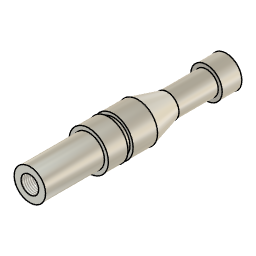
MSE 480 Lab 2 v4 (Autodesk Fusion 360 design; units mm, degrees)
Autodesk Fusion 360 part; units mm, degrees
note: some values were not read from the file. Chosen so that the rebuilt part matches the saved one: that a step has no effect; how an offset face is resized. Set by a fixed rule: which sketch regions a step uses.
sketch "Sketch2" plane through (0, 0, 0) normal (1, 0, 0) x (0, 1, 0)
  line L0 (0, 10.16) -> (38.1, 10.16)
  line L1 (38.1, 10.16) -> (38.1, 12.7)
  line L2 (38.1, 12.7) -> (50.8, 12.7)
  line L3 (50.8, 12.7) -> (50.8, 10.668)
  line L4 (50.8, 10.668) -> (54.102, 10.668)
  line L5 (54.102, 10.668) -> (54.102, 12.7)
  line L6 (54.102, 12.7) -> (69.9412, 12.7)
  line L7 (0, 10.16) -> (0, 0)
  line L8 (127, 0) -> (127, 10.16)
  line L9 (127, 10.16) -> (114.3, 10.16)
  line L10 (114.3, 10.16) -> (114.3, 7.62)
  line L11 (114.3, 7.62) -> (88.9, 7.62)
  line L12 (88.9, 7.62) -> (69.9412, 12.7)
  line L13 (0, 0) -> (127, 0)
  dimension "d4" = 3.302
  dimension "d5" = 12.7
  dimension "d6" = 38.1
  dimension "d14" = 127
  dimension "d15" = 25.4
  dimension "d16" = 12.7
  dimension "d17" = 2.54
  dimension "d30" = 165
  dimension "d64" = 10.16
  dimension "d65" = 10.16
  dimension "d72" = 2.032
  dimension "d73" = 2.54
  dimension "d74" = 7.62
  constraint perpendicular L0 L1
  constraint perpendicular L1 L2
  constraint perpendicular L2 L3
  constraint perpendicular L3 L4
  constraint perpendicular L4 L5
  constraint perpendicular L5 L6
  constraint perpendicular L0 L7
  constraint perpendicular L6 L8
  constraint perpendicular L8 L9
  constraint perpendicular L9 L10
  constraint perpendicular L8 L11
  constraint coincident L7.end L13.start
  constraint perpendicular L8 L13
  constraint coincident L13 L7.end
  measures "d4" distance of L3.end L4.end
  measures "d5" distance of L1.end L2.end
  measures "d6" distance of L0.start L0.end
  measures "d14" distance of L7 L8
  measures "d15" distance of L10.end L11.end
  measures "d16" distance of L8.end L9.end
  measures "d17" distance of L9.end L10.end
  measures "d30" angle of L6 L12
  measures "d64" distance of L0.start L7.end
  measures "d65" distance of L8.end L8.start
  measures "d72" distance of L2.end L3.end
  measures "d73" distance of L0.end L1.end
  measures "d74" distance of L11 L13
extrude "Extrude3" add sketch "Sketch2" along normal blind 25.4 makes body 1
delete_body "RemoveBody1" bodies 1
extrude "Extrude7" [no effect]
extrude "Extrude8" [no effect]
sketch "Sketch6" plane through (0, 0, 0) normal (0, -1, 0) x (1, 0, 0)
  circle A0 centre (0, 0) radius 10.16
  circle A1 centre (0, 0) radius 6.35
  dimension "d67" = 12.7
  constraint coincident A0.centre A1.centre
  measures "d67" diameter of A1
revolve "Revolve2" add sketch "Sketch2" angle 360 about axis through (0, 0, 0) along (0, 1, 0) separate body makes body 2
extrude "Extrude14" cut sketch "Sketch6" against normal blind 25.4 contours A1 bodies 2
thread "Thread2" "ANSI Unified Screw Threads 0.5 1/2-20 UNF 3B" major diameter 12.7 minor diameter 11.4275 pitch 1.27 angle 60 resizes the face on face at (6.3184, 16.9333, -0.6323) on bodies 2
